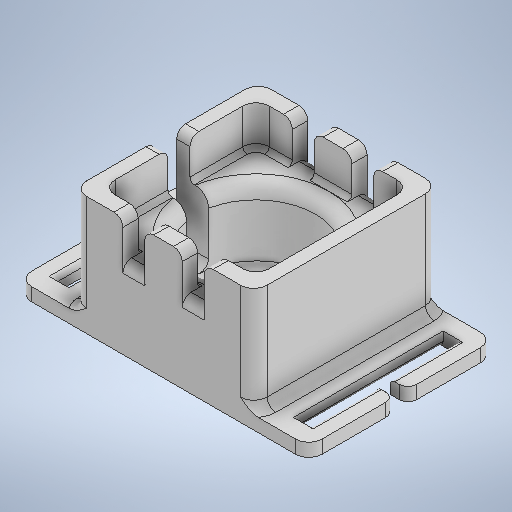
# Autodesk Inventor part: Strap Mount 1
Saved by Autodesk Inventor 2025 (Build 290162000, 162)
## iProperties
Created: 2024-12-27
Part Number: Strap Mount 1
Material: Generic
Document SubType Name: Modeling
Designer: Fahrul Ramadhan Putr
Density: 1 g/cm^3
Appearance: Default
Author: Fahrul Ramadhan Putr
Autodesk Inventor part; units mm, degrees
ref_plane "YZ Plane" through (0, 0, 0) normal (1, 0, 0) x (0, 1, 0)
ref_plane "XZ Plane" through (0, 0, 0) normal (0, 1, 0) x (-1, 0, 0)
ref_plane "XY Plane" through (0, 0, 0) normal (0, 0, 1) x (1, 0, 0)
sketch "Sketch1" plane through (0, 0, 0) normal (0, 1, 0) x (-1, 0, 0)
  line L0 (0, 0) -> (41, 0)
  line L1 (41, 0) -> (41, -42)
  line L2 (41, -42) -> (0, -42)
  line L3 (0, -42) -> (0, 0)
  circle A0 centre (20.5, -21) radius 13.5
  line L4 (41, 0) -> (53.5, 0)
  line L5 (53.5, 0) -> (53.5, -42)
  line L6 (53.5, -42) -> (41, -42)
  line L7 (41, -42) -> (41, 0)
  line L8 (41, -21) -> (53.5, -21)
  line L9 (53.5, -21) -> (53.5, -22.5)
  line L10 (53.5, -22.5) -> (41, -22.5)
  line L11 (41, -22.5) -> (41, -21)
  line L12 (41, -21) -> (53.5, -21)
  line L13 (53.5, -21) -> (53.5, -19.5)
  line L14 (53.5, -19.5) -> (41, -19.5)
  line L15 (41, -19.5) -> (41, -21)
  line L16 (41, 0) -> (53.5, 0)
  line L17 (53.5, 0) -> (53.5, -4)
  line L18 (53.5, -4) -> (41, -4)
  line L19 (41, -4) -> (41, 0)
  line L20 (53.5, -42) -> (41, -42)
  line L21 (41, -42) -> (41, -38)
  line L22 (41, -38) -> (53.5, -38)
  line L23 (53.5, -38) -> (53.5, -42)
  line L24 (53.5, 0) -> (49.5, 0)
  line L25 (49.5, 0) -> (49.5, -42)
  line L26 (49.5, -42) -> (53.5, -42)
  line L27 (53.5, -42) -> (53.5, 0)
  line L28 (0, 0) -> (-12.5, 0)
  line L29 (-12.5, 0) -> (-12.5, -42)
  line L30 (-12.5, -42) -> (0, -42)
  line L31 (0, -42) -> (0, 0)
  line L32 (0, -21) -> (-12.5, -21)
  line L33 (-12.5, -21) -> (-12.5, -19.5)
  line L34 (-12.5, -19.5) -> (0, -19.5)
  line L35 (0, -19.5) -> (0, -21)
  line L36 (0, -21) -> (-12.5, -21)
  line L37 (-12.5, -21) -> (-12.5, -22.5)
  line L38 (-12.5, -22.5) -> (0, -22.5)
  line L39 (0, -22.5) -> (0, -21)
  line L40 (0, 0) -> (-12.5, 0)
  line L41 (-12.5, 0) -> (-12.5, -4)
  line L42 (-12.5, -4) -> (0, -4)
  line L43 (0, -4) -> (0, 0)
  line L44 (0, -42) -> (-12.5, -42)
  line L45 (-12.5, -42) -> (-12.5, -38)
  line L46 (-12.5, -38) -> (0, -38)
  line L47 (0, -38) -> (0, -42)
  line L48 (-12.5, -42) -> (-8.5, -42)
  line L49 (-8.5, -42) -> (-8.5, 0)
  line L50 (-8.5, 0) -> (-12.5, 0)
  line L51 (-12.5, 0) -> (-12.5, -42)
  line L52 (38, -3.5) -> (3, -3.5)
  line L53 (3, -3.5) -> (3, -38.5)
  line L54 (3, -38.5) -> (38, -38.5)
  line L55 (38, -38.5) -> (38, -3.5)
  line L56 (41, -23) -> (41, -19.5)
  line L57 (0, 0) -> (-5, 0)
  line L58 (-5, 0) -> (-5, -42)
  line L59 (-5, -42) -> (0, -42)
  line L60 (0, -42) -> (0, 0)
  line L61 (41, 0) -> (46, 0)
  line L62 (46, 0) -> (46, -42)
  line L63 (46, -42) -> (41, -42)
  line L64 (41, -42) -> (41, 0)
  line L65 (41, -21) -> (33.7665, -21)
  line L66 (33.7665, -21) -> (33.7665, -23.5)
  line L67 (33.7665, -23.5) -> (41, -23.5)
  line L68 (41, -23.5) -> (41, -21)
  line L69 (41, -21) -> (33.7665, -21)
  line L70 (33.7665, -21) -> (33.7665, -18.5)
  line L71 (33.7665, -18.5) -> (41, -18.5)
  line L72 (41, -18.5) -> (41, -21)
  point P0 (46, -4)
  point P1 (49.5, -4)
  point P2 (49.5, -19.5)
  point P3 (-8.5, -19.5)
  point P4 (-8.5, -4)
  point P5 (-5, -4)
  point P6 (-5, -38)
  point P7 (-8.5, -38)
  point P8 (-8.5, -22.5)
  point P9 (0, -42)
  point P10 (49.5, -22.5)
  point P11 (49.5, -38)
  point P12 (46, -38)
  point P13 (38, -23.5)
  point P14 (38, -18.5)
  point P15 (41, -23.5)
  point P16 (41, -18.5)
  dimension "d0" = 41
  dimension "d1" = 42
  dimension "d2" = 27
  dimension "d3" = 12.5
  dimension "d4" = 1.5
  dimension "d5" = 1.5
  dimension "d6" = 4
  dimension "d7" = 4
  dimension "d8" = 4
  dimension "d9" = 12.5
  dimension "d10" = 1.5
  dimension "d11" = 1.5
  dimension "d12" = 4
  dimension "d13" = 4
  dimension "d14" = 4
  dimension "d15" = 35
  dimension "d16" = 35
  dimension "d17" = 3.5
  dimension "d18" = 3
  dimension "d23" = 5
  dimension "d24" = 5
  dimension "d36" = 42
  dimension "d37" = 42
  dimension "d38" = 2.5
  constraints: 146 end point, 36 parallel, 18 horizontal, 18 perpendicular, 13 point on line, 2 midpoint, 2 point on circle, 1 centre point
  measures "d0" distance of L1.end L2.end
  measures "d1" distance of L0.end L1.end
  measures "d2" diameter of A0
  measures "d3" distance of L5.end L6.end
  measures "d4" distance of L8.end L9.end
  measures "d5" distance of L13.end L12.end
  measures "d6" distance of L16.end L17.end
  measures "d7" distance of L20.end L21.end
  measures "d8" distance of L26.end L25.end
  measures "d9" distance of L30.end L29.end
  measures "d10" distance of L32.end L33.end
  measures "d11" distance of L37.end L36.end
  measures "d12" distance of L41.end L40.end
  measures "d13" distance of L44.end L45.end
  measures "d14" distance of L50.end L49.end
  measures "d15" distance of L54.end L53.end
  measures "d16" distance of L53.end L52.end
  measures "d17" distance between parallel lines of L52 L0
  measures "d18" distance between parallel lines of L55 L1
  measures "d23" distance of L59.end L58.end
  measures "d24" distance of L62.end L63.end
  measures "d36" distance between parallel lines of L30 L28
  measures "d37" distance between parallel lines of L6 L16
  measures "d38" distance between parallel lines of L65 L71
extrude "Extrusion1" add sketch "Sketch1" along normal blind 15 contours L71 A0 L67 L55 L54 L53 L52
extrude "Extrusion2" add sketch "Sketch1" along normal blind 24 contours L0 L1 L71 L55 L52 L53 L54 L67 L2 L3
extrude "Extrusion3" add sketch "Sketch1" against normal blind 3 contours L0 L1 L71 L55 L52 L53 L54 L67 L2 L3 | L3 L42 L58 L28 | L4 L62 L18 L1 | L3 L34 L58 L42 | L58 L42 L49 L28 | L18 L62 L14 L1 | L4 L25 L18 L62 | L3 L32 L58 L34 | L49 L42 L29 L28 | L1 L65 L55 L71 | L4 L5 L18 L25 | L3 L38 L58 L32 | L49 L34 L29 L42 | L14 L62 L8 L1 | L71 A0 L67 L55 L54 L53 L52 | L55 L65 A0 L71 | L18 L5 L14 L25 | L3 L46 L58 L38 | L8 L62 L10 L1 | L1 L67 L55 L65 | L55 L67 A0 L65 | L70 L66 A0 | A0 L65 L70 | L3 L30 L58 L46 | L10 L62 L22 L1 | A0 L66 L65 | L58 L30 L49 L46 | L49 L46 L29 L38 | L10 L5 L22 L25 | L62 L6 L1 L22 | L22 L25 L6 L62 | L49 L30 L29 L46 | L22 L5 L6 L25
fillet "Fillet1" radius 3 13 edges at (-41, 12, -42) (-41, 12, 0) (0, 12, 0) (0, 12, -42) (-38, 19.5, -3.5) (-38, 19.5, -38.5) (-3, 19.5, -38.5) (-3, 19.5, -3.5) (-7, 15, -21) (-53.5, -1.5, -42) (-53.5, -1.5, 0) (12.5, -1.5, -42) (12.5, -1.5, 0)
fillet "Fillet3" radius 1 6 edges at (5, -3, -21) (8.5, 0, -11.75) (8.5, 0, -30.25) (-46, -3, -21) (-49.5, 0, -30.25) (-49.5, 0, -11.75)
fillet "Fillet4" radius 2 11 edges at (12.5, -1.5, -22.5) (12.5, -1.5, -19.5) (-53.5, -1.5, -22.5) (-53.5, -1.5, -19.5) (-40.1213, 0, -0.8787) (-41, 0, -10.75) (-40.1213, 0, -41.1213) (-41, 0, -31.25) (0, 0, -21) (-0.8787, 0, -41.1213) (-0.8787, 0, -0.8787)
sketch "Sketch4" plane through (0, 15, 0) normal (0, 1, 0) x (1, 0, 0)
  arc A0 (0, 39) -> (-3, 42) centre (-3, 39) ccw projected
  line L0 (-3, 42) -> (-38, 42) projected
  arc A1 (-38, 42) -> (-41, 39) centre (-38, 39) ccw projected
  line L1 (-41, 39) -> (-41, 23.5) projected
  line L2 (-41, 23.5) -> (-38, 23.5) projected
  line L3 (-38, 23.5) -> (-38, 35.5) projected
  arc A2 (-35, 38.5) -> (-38, 35.5) centre (-35, 35.5) ccw projected
  line L4 (-35, 38.5) -> (-6, 38.5) projected
  arc A3 (-3, 35.5) -> (-6, 38.5) centre (-6, 35.5) ccw projected
  line L5 (-3, 35.5) -> (-3, 6.5) projected
  arc A4 (-6, 3.5) -> (-3, 6.5) centre (-6, 6.5) ccw projected
  line L6 (-6, 3.5) -> (-35, 3.5) projected
  arc A5 (-38, 6.5) -> (-35, 3.5) centre (-35, 6.5) ccw projected
  line L7 (-38, 6.5) -> (-38, 18.5) projected
  line L8 (-38, 18.5) -> (-41, 18.5) projected
  line L9 (-41, 18.5) -> (-41, 3) projected
  arc A6 (-41, 3) -> (-38, 0) centre (-38, 3) ccw projected
  line L10 (-38, 0) -> (-3, 0) projected
  arc A7 (-3, 0) -> (0, 3) centre (-3, 3) ccw projected
  line L11 (0, 3) -> (0, 39) projected
  line L12 (-20.5, 21) -> (-20.5, 0)
  line L13 (-20.5, 0) -> (-27.25, 0)
  line L14 (-38, 0) -> (-3, 0) projected
  line L15 (-20.5, 0) -> (-13.75, 0)
  line L16 (-13.75, 0) -> (-11.25, 0)
  line L17 (-27.25, 0) -> (-29.75, 0)
  line L18 (-11.25, 0) -> (-16.25, 0)
  line L19 (-16.25, 0) -> (-16.25, 42)
  line L20 (-16.25, 42) -> (-11.25, 42)
  line L21 (-11.25, 42) -> (-11.25, 0)
  line L22 (-29.75, 0) -> (-24.75, 0)
  line L23 (-24.75, 0) -> (-24.75, 42)
  line L24 (-24.75, 42) -> (-29.75, 42)
  line L25 (-29.75, 42) -> (-29.75, 0)
  point P0 (0, 0)
  point P1 (-11.25, 38.5)
  point P2 (-16.25, 38.5)
  point P3 (-29.75, 38.5)
  point P4 (-24.75, 38.5)
  point P5 (-29.75, 3.5)
  point P6 (-24.75, 3.5)
  point P7 (-11.25, 3.5)
  point P8 (-16.25, 3.5)
  dimension "d41" = 6.75
  dimension "d42" = 6.75
  dimension "d43" = 2.5
  dimension "d44" = 2.5
  dimension "d45" = 5
  dimension "d46" = 5
  constraints: 26 end point, 6 point on line, 4 parallel, 2 horizontal, 2 perpendicular, 1 midpoint
  measures "d41" distance of L12.end L13.end
  measures "d42" distance of L12.end L15.end
  measures "d43" distance of L15.end L16.end
  measures "d44" distance of L13.end L17.end
  measures "d45" distance of L19.end L20.end
  measures "d46" distance of L24.end L23.end
extrude "Extrusion6" cut sketch "Sketch4" along normal up to surface (9 mm away) contours L21 L4 L19 L0 | L10 L19 L6 L21 | L23 L4 L25 L0 | L23 L10 L25 L6
fillet "Fillet5" radius 2 16 edges at (-13.75, 15, 0) (-27.25, 15, 0) (-13.75, 15, -42) (-27.25, 15, -42) (-16.25, 24, -40.25) (-24.75, 24, -40.25) (-11.25, 24, -40.25) (-29.75, 24, -40.25) (-24.75, 24, -1.75) (-16.25, 24, -1.75) (-11.25, 24, -1.75) (-29.75, 24, -1.75) (-39.5, 24, -23.5) (-39.5, 24, -18.5) (-38.3832, 0, -23.5) (-38.3832, 0, -18.5)
fillet "Fillet6" radius 1 13 edges at (-20.5, 15, -38.5) (-37.1213, 15, -37.6213) (-38, 15, -29.5) (-32.375, 15, -38.5) (-3.8787, 15, -37.6213) (-3, 15, -21) (-3.8787, 15, -4.3787) (-8.625, 15, -3.5) (-8.625, 15, -38.5) (-20.5, 15, -3.5) (-37.1213, 15, -4.3787) (-38, 15, -12.5) (-32.375, 15, -3.5)
body "Solid1"
